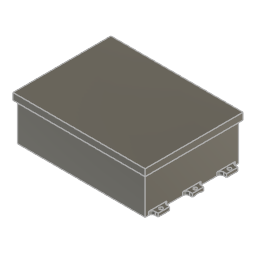
electronics holder2 (Autodesk Fusion 360 design; units mm, degrees)
part number: 2026-07-19-20-42-42-354
Autodesk Fusion 360 part; units mm, degrees
sketch "Sketch1" plane through (0, 0, 0) normal (0, 0, 1) x (1, 0, 0)
  line L0 (-45, 20) -> (55, 20)
  line L1 (55, 20) -> (55, -50)
  line L2 (55, -50) -> (-45, -50)
  line L3 (-45, -50) -> (-45, 20)
  dimension "d1" = 100
  dimension "d2" = 70
  constraint horizontal L0
  constraint vertical L1
  constraint horizontal L2
  constraint vertical L3
  measures "d1" distance of L0.start L0.end
  measures "d2" distance of L0.start L2.end
extrude "Extrude1" add sketch "Sketch1" along normal blind 21 makes body 1
sketch "Sketch2" plane through (0, 0, 0) normal (0, 0, 1) x (1, 0, 0)
  line L0 (-45, 20) -> (55, 20)
  line L1 (55, 20) -> (55, -50)
  line L2 (55, -50) -> (-45, -50)
  line L3 (-45, -50) -> (-45, 20)
  line L4 (-45, -50) -> (55, 20)
  line L5 (-45, 20) -> (55, -50)
  line L6 (61, 26) -> (-51, 26)
  line L7 (-51, 26) -> (-51, -56)
  line L8 (-51, -56) -> (61, -56)
  line L9 (61, -56) -> (61, 26)
  line L10 (61, 26) -> (-51, -56) construction
  line L11 (-51, 26) -> (61, -56) construction
  point P0 (5, -15)
  dimension "d5" = 112
  dimension "d6" = 82
  constraint horizontal L0
  constraint vertical L1
  constraint horizontal L2
  constraint vertical L3
  constraint horizontal L6
  constraint perpendicular L6 L7
  constraint parallel L6 L8
  constraint parallel L7 L9
  constraint coincident L10 P0
  constraint coincident L11 P0
  constraint midpoint L5 P0
  measures "d5" distance of L7.end L8.end
  measures "d6" distance of L6.end L7.end
extrude "Extrude2" add sketch "Sketch2" along normal blind 2 separate body contours L3 L4 L5 | L0 L4 L5 | L1 L4 L5 | L2 L4 L5 | L6 L7 L8 L9 makes body 2
sketch "Sketch3" plane through (0, 0, 2) normal (0, 0, 1) x (-1, 0, 0)
  line L0 (-61, 56) -> (-61, -26)
  line L1 (-61, -26) -> (51, -26)
  line L2 (51, -26) -> (51, 56)
  line L3 (51, 56) -> (-61, 56)
  line L4 (-61, -26) -> (51, 56)
  line L5 (-61, 56) -> (51, -26)
  line L6 (49, 54) -> (-59, 54)
  line L7 (-59, 54) -> (-59, -24)
  line L8 (-59, -24) -> (49, -24)
  line L9 (49, -24) -> (49, 54)
  line L10 (49, 54) -> (-59, -24) construction
  line L11 (-59, 54) -> (49, -24) construction
  point P0 (-5, 15)
  dimension "d9" = 108
  dimension "d10" = 78
  constraint coincident L0.end L1.start
  constraint coincident L2.end L3.start
  constraint coincident L0.start L3.end
  constraint coincident L1.end L2.start
  constraint horizontal L6
  constraint perpendicular L6 L7
  constraint parallel L6 L8
  constraint parallel L7 L9
  constraint coincident L10 P0
  constraint coincident L11 P0
  constraint midpoint L4 P0
  measures "d9" distance of L7.end L8.end
  measures "d10" distance of L6.end L7.end
extrude "Extrude3" add sketch "Sketch3" along normal blind 35 contours L0 L4 L5 L6 L7 L8 | L3 L4 L5 L6 | L1 L4 L5 L8 | L2 L4 L5 L6 L8 L9 bodies 2
move_body "Move1" bodies 1 to x (1, 0, 0) y (0, 1, 0) z (0, 0, 1) at (0, 0, 3)
sketch "Sketch4" plane through (0, 0, 37) normal (0, 0, 1) x (-1, 0, 0)
  line L0 (49, 54) -> (49, -24)
  line L1 (49, -24) -> (-59, -24)
  line L2 (-59, -24) -> (-59, 54)
  line L3 (-59, 54) -> (49, 54)
  line L4 (51, 56) -> (-61, 56)
  line L5 (-61, 56) -> (-61, -26)
  line L6 (-61, -26) -> (51, -26)
  line L7 (51, -26) -> (51, 56)
  line L8 (51, 56) -> (-61, -26)
  line L9 (51, -26) -> (-61, 56)
  line L10 (53, -28) -> (-63, -28)
  line L11 (-63, -28) -> (-63, 58)
  line L12 (-63, 58) -> (53, 58)
  line L13 (53, 58) -> (53, -28)
  line L14 (53, -28) -> (-63, 58) construction
  line L15 (-63, -28) -> (53, 58) construction
  line L16 (51, -26) -> (-61, -26)
  line L17 (-61, -26) -> (-61, 56)
  line L18 (-61, 56) -> (51, 56)
  line L19 (51, 56) -> (51, -26)
  line L20 (51, -26) -> (-61, 56) construction
  line L21 (-61, -26) -> (51, 56) construction
  point P0 (-5, 15)
  point P1 (-5, 15)
  dimension "d13" = 116
  dimension "d14" = 86
  constraint coincident L4.start L7.end
  constraint coincident L5.end L6.start
  constraint coincident L6.end L7.start
  constraint coincident L4.end L5.start
  constraint horizontal L10
  constraint perpendicular L10 L11
  constraint parallel L10 L12
  constraint parallel L11 L13
  constraint coincident L14 P1
  constraint coincident L15 P1
  constraint midpoint L8 P1
  constraint horizontal L16
  constraint perpendicular L16 L17
  constraint parallel L16 L18
  constraint parallel L17 L19
  constraint coincident L20 P1
  constraint coincident L21 P1
  constraint coincident P1 P0
  measures "d13" distance of L11.end L12.end
  measures "d14" distance of L10.end L11.end
extrude "Extrude4" add sketch "Sketch4" along normal blind 2 separate body contours L0 L1 L3 L7 L8 L9 L19 | L0 L1 L3 L8 L9 | L3 L8 L9 | L3 L4 L8 L9 L18 | L1 L6 L8 L9 L16 | L1 L8 L9 | L1 L2 L3 L8 L9 | L1 L2 L3 L5 L8 L9 L17 | L10 L11 L12 L13 makes body 3
sketch "Sketch5" plane through (0, 0, 37) normal (0, 0, -1) x (1, 0, 0)
  line L0 (63, 58) -> (-53, 58)
  line L1 (-53, 58) -> (-53, -28)
  line L2 (-53, -28) -> (63, -28)
  line L3 (63, -28) -> (63, 58)
  line L4 (-53, 58) -> (63, 58)
  line L5 (63, 58) -> (63, -28)
  line L6 (63, -28) -> (-53, -28)
  line L7 (-53, -28) -> (-53, 58)
  line L8 (-53, 58) -> (63, -28) construction
  line L9 (-51.5, 56.5) -> (61.5, 56.5)
  line L10 (61.5, 56.5) -> (61.5, -26.5)
  line L11 (61.5, -26.5) -> (-51.5, -26.5)
  line L12 (-51.5, -26.5) -> (-51.5, 56.5)
  point P0 (5, 15)
  point P1 (5, 15)
  dimension "d17" = 113
  dimension "d18" = 83
  constraint horizontal L4
  constraint perpendicular L4 L5
  constraint parallel L4 L6
  constraint parallel L5 L7
  constraint coincident L8 P1
  constraint coincident L0.end L1.start
  constraint horizontal L9
  constraint perpendicular L9 L10
  constraint parallel L9 L11
  constraint parallel L10 L12
  constraint coincident P1 P0
  measures "d17" distance of L10.end L11.end
  measures "d18" distance of L9.end L10.end
extrude "Extrude5" add sketch "Sketch5" along normal blind 8 bodies 3
extrude "Extrude6" cut 1 faces at (23.8333, 27.5, 29) along direction (0, 0, 1) blind 4 on bodies 3 bodies 3
sketch "Sketch6" plane through (0, 0, 0) normal (0, 0, -1) x (1, 0, 0)
  line L0 (61, -26) -> (61, 56)
  line L1 (61, 56) -> (-51, 56)
  line L2 (-51, 56) -> (-51, -26)
  line L3 (-51, -26) -> (61, -26)
  line L4 (-51, 56) -> (61, -26)
  line L5 (-51, -26) -> (61, 56)
  line L6 (66.5, 20) -> (-56.5, 20)
  line L7 (-56.5, 20) -> (-56.5, 10)
  line L8 (-56.5, 10) -> (66.5, 10)
  line L9 (66.5, 10) -> (66.5, 20)
  line L10 (66.5, 20) -> (-56.5, 10) construction
  line L11 (-56.5, 20) -> (66.5, 10) construction
  circle A0 centre (-54, 15) radius 1.5
  circle A1 centre (64, 15) radius 1.5
  line L12 (5, -15) -> (5, 45)
  line L13 (-56.5, 50) -> (66.5, 50)
  line L14 (66.5, 50) -> (66.5, 40)
  line L15 (66.5, 40) -> (-56.5, 40)
  line L16 (-56.5, 40) -> (-56.5, 50)
  line L17 (-56.5, 50) -> (66.5, 40) construction
  line L18 (66.5, 50) -> (-56.5, 40) construction
  line L19 (-56.5, -10) -> (66.5, -10)
  line L20 (66.5, -10) -> (66.5, -20)
  line L21 (66.5, -20) -> (-56.5, -20)
  line L22 (-56.5, -20) -> (-56.5, -10)
  line L23 (-56.5, -10) -> (66.5, -20) construction
  line L24 (66.5, -10) -> (-56.5, -20) construction
  line L25 (5, 15) -> (5, 45)
  line L26 (5, 15) -> (5, -15)
  line L27 (5, 0) -> (-4, 0)
  circle A2 centre (-54, -15) radius 1.5
  circle A3 centre (64, -15) radius 1.5
  line L28 (5, 30) -> (-15, 30)
  circle A4 centre (-54, 45) radius 1.5
  circle A5 centre (64, 45) radius 1.5
  point P0 (5, 15)
  point P1 (5, 15)
  point P2 (5, 15)
  point P3 (5, 45)
  point P4 (5, -15)
  dimension "d23" = 123
  dimension "d24" = 10
  dimension "d25" = 3
  dimension "d26" = 123
  dimension "d27" = 10
  dimension "d28" = 123
  dimension "d29" = 10
  constraint coincident L1.end L2.start
  constraint coincident L0.start L3.end
  constraint coincident L2.end L3.start
  constraint coincident L0.end L1.start
  constraint horizontal L6
  constraint perpendicular L6 L7
  constraint parallel L6 L8
  constraint parallel L7 L9
  constraint coincident L10 P2
  constraint coincident L11 P2
  constraint midpoint L4 P2
  constraint coincident P2 P1
  constraint midpoint L12 P2
  constraint vertical L12
  constraint horizontal L13
  constraint perpendicular L13 L14
  constraint parallel L13 L15
  constraint parallel L14 L16
  constraint coincident L17 P3
  constraint coincident L18 P3
  constraint coincident P3 L12.end
  constraint horizontal L19
  constraint perpendicular L19 L20
  constraint parallel L19 L21
  constraint parallel L20 L22
  constraint coincident L23 P4
  constraint coincident L24 P4
  constraint coincident P4 L12.start
  constraint midpoint L26 L27.start
  constraint perpendicular L12 L27
  constraint symmetric A0 L27 A2
  constraint symmetric A1 L27 A3
  constraint midpoint L25 L28.start
  constraint perpendicular L12 L28
  constraint symmetric A0 L28 A4
  constraint symmetric A1 L28 A5
  measures "d23" distance of L7.end L8.end
  measures "d24" distance of L6.end L7.end
  measures "d25" diameter of A0
  measures "d26" distance of L14.end L15.end
  measures "d27" distance of L13.end L14.end
  measures "d28" distance of L20.end L21.end
  measures "d29" distance of L19.end L20.end
extrude "Extrude7" add sketch "Sketch6" against normal blind 3 contours L0 L19 L20 L21 | L2 L19 L21 L22 | L0 L6 L8 L9 | L2 L6 L7 L8 | L0 L13 L14 L15 | L2 L13 L15 L16 bodies 2
fillet "Fillet1" radius 3 13 edges at (62.6015, -15.5424, 0) (61, -10, 1.5) (61, 20, 1.5) (61, -40, 1.5) (61, -50, 1.5) (61, -20, 1.5) (61, 10, 1.5) (-51, -50, 1.5) (-51, -20, 1.5) (-51, 10, 1.5) (-51, 20, 1.5) (-51, -40, 1.5) (-51, -10, 1.5) on bodies 2
named bodies: "odrive bottom casing shell", "top casing lid"
